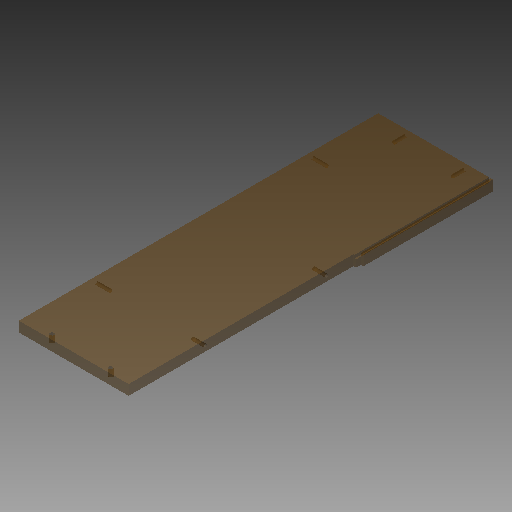
# Autodesk Inventor part: Wand2
Saved by Autodesk Inventor 2018 (Build 220112000, 112)
## iProperties
Created: 2013-02-21
Part Number: Wand2
Material: Polycarbonate, Smoke
Document SubType Name: Modeling
Designer: Neef
Mass: 172.08 g
Surface Area: 416.34 cm^2
Volume: 143.4 cm^3
Density: 1.2 g/cm^3
Appearance: Polycarbonate - Smoked
Author: Neef
Autodesk Inventor part; units mm, degrees
ref_plane "YZ Plane" through (0, 0, 0) normal (1, 0, 0) x (0, 1, 0)
ref_plane "XZ Plane" through (0, 0, 0) normal (0, 1, 0) x (-1, 0, 0)
ref_plane "XY Plane" through (0, 0, 0) normal (0, 0, 1) x (1, 0, 0)
sketch "Skizze1" plane through (0, 0, 0) normal (0, 0, 1) x (1, 0, 0)
  line L0 (45, 140.75) -> (-45, 140.75)
  line L1 (-45, 140.75) -> (-45, -140.75)
  line L2 (-45, -140.75) -> (45, -140.75)
  line L3 (45, -140.75) -> (45, 140.75)
  line L4 (0, 197.05) -> (0, -197.05) projected
  line L5 (-63, 0) -> (63, 0) projected
  point P0 (0, 0)
  point P1 (45, 0)
  point P2 (0, -140.75)
  dimension "d0" = 281.5
  dimension "d1" = 90
  constraints: 8 end point, 2 midpoint, 2 parallel, 2 point on line, 1 horizontal, 1 perpendicular
  measures "d0" distance of L2.end L0.start
  measures "d1" distance of L1.end L2.end
extrude "Extrusion1" add sketch "Skizze1" along normal blind 8
sketch "Skizze2" plane through (-45, -140.75, 0) normal (0, -1, 0) x (1, 0, 0)
  line L0 (90, 8) -> (0, 8) projected
  line L1 (86.8, 8) -> (88, 8)
  line L2 (88, 8) -> (88, 5.5)
  line L3 (88, 5.5) -> (86.8, 5.5)
  line L4 (86.8, 5.5) -> (86.8, 8)
  line L5 (90, 0) -> (90, 8) projected
  point P0 (45, 0)
  dimension "d4" = 1.2
  dimension "d5" = 2.5
  dimension "d8" = 2
  constraints: 8 end point, 2 parallel, 1 horizontal, 1 perpendicular, 1 point on line
  measures "d4" distance of L2.end L3.end
  measures "d5" distance of L1.end L2.end
  measures "d8" distance between parallel lines of L5 L2
extrude "Extrusion2" cut sketch "Skizze2" against normal through all
sketch "Skizze3" plane through (0, 0, 0) normal (0, 0, -1) x (-1, 0, 0)
  line L0 (-45, -140.75) -> (-41, -140.75)
  line L1 (-41, -140.75) -> (-41, 39.25)
  line L2 (-41, 39.25) -> (-45, 39.25)
  line L3 (-45, 39.25) -> (-45, -140.75)
  point P0 (0, 0)
  dimension "d9" = 4
  dimension "d10" = 180
  constraints: 8 end point, 2 parallel, 1 horizontal, 1 perpendicular
  measures "d9" distance of L1.end L2.end
  measures "d10" distance of L0.end L1.end
extrude "Extrusion3" cut sketch "Skizze3" against normal through all
sketch "Skizze4" plane through (0, 0, 0) normal (0, 0, -1) x (-1, 0, 0)
  line L0 (-41, 39.25) -> (-43, 39.25)
  line L1 (-43, 39.25) -> (-43, 35.25)
  line L2 (-43, 35.25) -> (-41, 35.25)
  line L3 (-41, 35.25) -> (-41, 39.25)
  point P0 (0, 0)
  dimension "d13" = 4
  dimension "d14" = 2
  constraints: 8 end point, 2 parallel, 1 horizontal, 1 perpendicular
  measures "d13" distance of L0.end L1.end
  measures "d14" distance of L1.end L2.end
extrude "Extrusion4" add sketch "Skizze4" against normal blind 5.5
sketch "Skizze5" plane through (41.8, 39.25, 5.5) normal (0, 0, 1) x (1, 0, 0)
  line L0 (0, 0) -> (-0.8, 0)
  line L1 (-0.8, 0) -> (-0.8, -4)
  line L2 (-0.8, -4) -> (0, -4)
  line L3 (0, -4) -> (0, 0)
  point P0 (-41.8, -39.25)
  constraints: 8 end point, 2 parallel, 1 horizontal, 1 perpendicular
extrude "Extrusion5" add sketch "Skizze5" along normal up to surface (2.5 mm away)
sketch "Skizze6" plane through (-45, -140.75, 0) normal (-1, 0, 0) x (0, 0, 1)
  line L0 (0, 0) -> (8, 0) projected
  line L1 (0, 281.5) -> (8, 281.5) projected
  line L2 (0, 281.5) -> (0, 0) projected
  point P0 (0, 140.75)
  point P1 (4, 60)
  point P2 (4, 229.5)
  dimension "d19" = 60
  dimension "d41" = 52
  dimension "d42" = 4
  measures "d19" distance from line of point (4, 60) L0
  measures "d41" distance from line of L1 point (4, 229.5)
  measures "d42" distance from line of L2 point (4, 229.5)
hole "Bohrung1" at (-45, -80.75, 4) at (-45, 88.75, 4) direction (1, 0, 0) diameter 2.459 depth 12 tip angle 118 thread size "M3x0.5" class "6H" standard "ISO Metric profile"
sketch "Skizze7" plane through (-45, 140.75, 0) normal (0, 1, 0) x (1, 0, 0)
  arc A0 (90, -95.2303) -> (67.5, -77) centre (67.5, -100) ccw projected
  line L0 (90, 0) -> (90, -95.2303) projected
  line L1 (0, 0) -> (90, 0) projected
  line L2 (0, -77) -> (0, 0) projected
  line L3 (0, -77) -> (67.5, -77) projected
  point P0 (22, -4)
  point P1 (68, -4)
hole "Bohrung2" at (-23, 140.75, 4) at (23, 140.75, 4) direction (0, -1, 0) diameter 2.459 depth 10 tip angle 118 thread size "M3x0.5" class "6H" standard "ISO Metric profile"
sketch "Skizze8" plane through (0, 0, 0) normal (0, 0, -1) x (-1, 0, 0)
  line L0 (-41.8, 35.25) -> (-41.8, 140.75) projected
  line L1 (45, 140.75) -> (-41.8, 140.75) projected
  line L2 (45, -140.75) -> (45, 140.75) projected
  line L3 (-41, -140.75) -> (45, -140.75) projected
  line L4 (-41, -140.75) -> (-41, 35.25) projected
  line L5 (-41.8, 35.25) -> (-41, 35.25) projected
  circle A0 centre (-23, -136.75) radius 3.1 projected
  circle A1 centre (23, -136.75) radius 3.1 projected
  line L6 (45, -140.75) -> (45, 140.75) projected
  line L7 (-41, -140.75) -> (45, -140.75) projected
  line L8 (-41, 140.75) -> (-41, -140.75) projected
  line L9 (45, 140.75) -> (-41, 140.75) projected
  point P0 (0, 0)
  constraints: 2 coincident
hole "Bohrung3" at (23, -136.75, 0) at (-23, -136.75, 0) direction (0, 0, 1) diameter 3.2 end through all countersink diameter 6.2 countersink angle 90
sketch "Skizze10" plane through (41, -140.75, 8) normal (1, 0, 0) x (0, 0, -1)
  circle A0 centre (4, 155) radius 3.1 projected
  circle A1 centre (4, 60) radius 3.1 projected
  point P0 (8, 140.75)
  constraints: 2 coincident
hole "Bohrung4" at (41, -80.75, 4) at (41, 14.25, 4) direction (-1, 0, 0) diameter 2.459 depth 10 tip angle 118 thread size "M3x0.5" class "6H" standard "ISO Metric profile"
